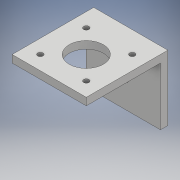
# Autodesk Inventor part: non_motor_holder
Saved by Autodesk Inventor 2017 (Build 210142000, 142)
## iProperties
Part Number: non_motor_holder
Material: Типовые
Document SubType Name: Modeling
Designer: Tolya
Density: 1 g/cm^3
Appearance: По умолчанию
Author: Tolya
Autodesk Inventor part; units mm, degrees
ref_plane "YZ Plane" through (0, 0, 0) normal (1, 0, 0) x (0, 1, 0)
ref_plane "XZ Plane" through (0, 0, 0) normal (0, 1, 0) x (-1, 0, 0)
ref_plane "XY Plane" through (0, 0, 0) normal (0, 0, 1) x (1, 0, 0)
sketch "Эскиз1" plane through (0, 0, 0) normal (0, 0, 1) x (1, 0, 0)
  line L0 (-25, -25) -> (25, -25)
  line L1 (25, -25) -> (25, 25)
  line L2 (25, 25) -> (-25, 25)
  line L3 (-25, 25) -> (-25, -25)
  circle A0 centre (0, 0) radius 11.5
  circle A1 centre (15.5, 15.5) radius 1.8
  circle A2 centre (-15.5, 15.5) radius 1.8
  circle A3 centre (-15.5, -15.5) radius 1.8
  circle A4 centre (15.5, -15.5) radius 1.8
  dimension "d0" = 50
  dimension "d1" = 50
  dimension "d2" = 23
  dimension "d3" = 3.6
  dimension "d6" = 360
  dimension "d14" = 25
  dimension "d15" = 25
  dimension "d16" = 9.5
  dimension "d17" = 9.5
  constraints: 8 end point, 5 centre point, 2 parallel, 1 coincident, 1 horizontal, 1 perpendicular, 9 other
  measures "d0" distance of L2.end L1.end
  measures "d1" distance of L1.end L0.end
  measures "d2" diameter of A0
  measures "d3" diameter of A1
  measures "d14" distance from line of point (0, 0) L1
  measures "d15" distance from line of point (0, 0) L2
  measures "d16" distance from line of A1.centre L1
  measures "d17" distance from line of A1.centre L2
extrude "Выдавливание1" add sketch "Эскиз1" along normal blind 5
sketch "Эскиз2" plane through (-25, 25, 0) normal (0, 1, 0) x (1, 0, 0)
  line L0 (0, 0) -> (50, 0)
  line L1 (50, 0) -> (50, 39)
  line L2 (50, 39) -> (0, 39)
  line L3 (0, 39) -> (0, 0)
  line L4 (0, -5) -> (50, -5) projected
  line L5 (50, 0) -> (50, -5) projected
  line L6 (0, -5) -> (50, -5)
  line L7 (50, -5) -> (50, 0)
  line L8 (50, 0) -> (0, 0)
  line L9 (0, 0) -> (0, -5)
  circle A0 centre (25, 19.5) radius 4.05
  point P0 (25, 0)
  dimension "d10" = 50
  dimension "d11" = 39
  dimension "d19" = 8.1
  constraints: 16 end point, 4 parallel, 2 horizontal, 2 perpendicular, 1 centre point
  measures "d10" distance of L2.end L1.end
  measures "d11" distance of L1.end L0.end
  measures "d19" diameter of A0
extrude "Выдавливание3" add sketch "Эскиз2" along normal blind 5
